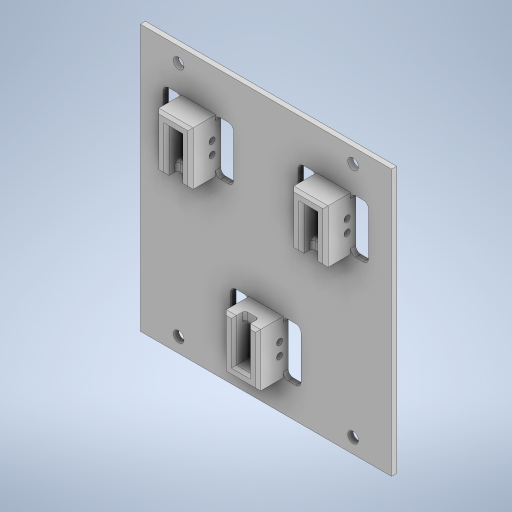
# Autodesk Inventor part: 01EjectionPlate
Saved by Autodesk Inventor 2023 (Build 270158000, 158)
## iProperties
Created: 2023-02-07
Part Number: 01EjectionPlate
Material: Generic
Document SubType Name: Modeling
Designer: 17038
Density: 1 g/cm^3
Appearance: Default
Author: 17038
Autodesk Inventor part; units mm, degrees
ref_plane "YZ Plane" through (0, 0, 0) normal (1, 0, 0) x (0, 1, 0)
ref_plane "XZ Plane" through (0, 0, 0) normal (0, 1, 0) x (-1, 0, 0)
ref_plane "XY Plane" through (0, 0, 0) normal (0, 0, 1) x (1, 0, 0)
sketch "Sketch1" plane through (0, 0, 0) normal (0, 0, 1) x (1, 0, 0)
  line L0 (-49.085, -51.99) -> (49.085, -51.99)
  line L1 (49.085, -51.99) -> (49.085, 51.99)
  line L2 (49.085, 51.99) -> (-49.085, 51.99)
  line L3 (-49.085, 51.99) -> (-49.085, -51.99)
  line L4 (-49.085, -51.99) -> (49.085, 51.99) construction
  line L5 (49.085, -51.99) -> (-49.085, 51.99) construction
  point P0 (0, 0)
  dimension "d0" = 103.98
  dimension "d1" = 98.17
  constraints: 12 end point, 2 midpoint, 2 parallel, 1 horizontal, 1 perpendicular
  measures "d0" distance of L0.end L1.end
  measures "d1" distance of L1.end L2.end
extrude "Extrusion1" add sketch "Sketch1" along normal blind 2
sketch "Sketch2" plane through (0, 0, 2) normal (0, 0, 1) x (1, 0, 0)
  line L0 (49.085, 51.99) -> (-49.085, 51.99) projected
  line L1 (-49.085, 51.99) -> (-49.085, -51.99) projected
  circle A0 centre (-34.085, 46.25) radius 2.05
  line L2 (-49.085, -51.99) -> (49.085, -51.99) construction
  line L3 (0, 51.99) -> (0, -51.99) construction
  circle A1 centre (34.085, 46.25) radius 2.05
  circle A2 centre (-34.085, -46.27) radius 2.05
  circle A3 centre (34.085, -46.27) radius 2.05
  point P0 (0, 0)
  dimension "d4" = 4.1
  dimension "d5" = 5.74
  dimension "d6" = 15
  dimension "d9" = 4.1
  dimension "d10" = 15
  dimension "d11" = 5.72
  constraints: 4 centre point, 2 end point, 2 midpoint, 2 symmetric about line, 2 other
  measures "d4" diameter of A0
  measures "d5" distance from line of L0 A0.centre
  measures "d6" distance from line of L1 A0.centre
  measures "d9" diameter of A2
  measures "d10" distance from line of L1 A2.centre
  measures "d11" distance from line of L2 A2.centre
extrude "Extrusion2" cut sketch "Sketch2" against normal up to surface (2 mm away)
sketch "Sketch4" plane through (0, 0, 2) normal (0, 0, 1) x (1, 0, 0)
  line L0 (49.085, -51.99) -> (49.085, 51.99) projected
  line L1 (49.085, 51.99) -> (-49.085, 51.99) projected
  line L2 (-49.085, 51.99) -> (-49.085, -51.99) projected
  line L3 (-49.085, -51.99) -> (49.085, -51.99) projected
  line L4 (-29.085, 19.19) -> (-23.685, 19.19)
  line L5 (-23.685, 19.19) -> (-23.685, 31.99)
  line L6 (-23.685, 31.99) -> (-29.085, 31.99)
  line L7 (-29.085, 31.99) -> (-29.085, 19.19)
  line L8 (-33.085, 15.19) -> (-19.685, 15.19)
  line L9 (-19.685, 15.19) -> (-19.685, 35.99)
  line L10 (-19.685, 35.99) -> (-33.085, 35.99)
  line L11 (-33.085, 35.99) -> (-33.085, 15.19)
  line L12 (0, 51.99) -> (0, -51.99) construction
  line L13 (29.085, 19.19) -> (23.685, 19.19)
  line L14 (23.685, 19.19) -> (23.685, 31.99)
  line L15 (23.685, 31.99) -> (29.085, 31.99)
  line L16 (29.085, 31.99) -> (29.085, 19.19)
  line L17 (33.085, 15.19) -> (19.685, 15.19)
  line L18 (19.685, 15.19) -> (19.685, 35.99)
  line L19 (19.685, 35.99) -> (33.085, 35.99)
  line L20 (33.085, 35.99) -> (33.085, 15.19)
  line L21 (-49.085, 0) -> (49.085, 0) construction
  line L22 (-2.7, -35.8497) -> (2.7, -35.8497)
  line L23 (2.7, -35.8497) -> (2.7, -23.0497)
  line L24 (2.7, -23.0497) -> (-2.7, -23.0497)
  line L25 (-2.7, -23.0497) -> (-2.7, -35.8497)
  line L26 (-2.7, -35.8497) -> (2.7, -23.0497) construction
  line L27 (2.7, -35.8497) -> (-2.7, -23.0497) construction
  line L28 (-6.7, -39.8497) -> (6.7, -39.8497)
  line L29 (6.7, -39.8497) -> (6.7, -19.0497)
  line L30 (6.7, -19.0497) -> (-6.7, -19.0497)
  line L31 (-6.7, -19.0497) -> (-6.7, -39.8497)
  line L32 (-6.7, -39.8497) -> (6.7, -19.0497) construction
  line L33 (6.7, -39.8497) -> (-6.7, -19.0497) construction
  point P0 (0, 0)
  point P1 (-26.385, 19.19)
  point P2 (0, -29.4497)
  dimension "d12" = 5.4
  dimension "d13" = 12.8
  dimension "d14" = 20
  dimension "d15" = 20
  dimension "d16" = 4
  dimension "d17" = 4
  dimension "d18" = 4
  dimension "d19" = 4
  dimension "d20" = 12.8
  dimension "d21" = 5.4
  dimension "d22" = 4
  dimension "d23" = 4
  dimension "d24" = 4
  dimension "d25" = 4
  constraints: 60 end point, 9 midpoint, 8 parallel, 8 symmetric about line, 4 horizontal, 4 perpendicular, 1 point on line
  measures "d12" distance of L4.start L4.end
  measures "d13" distance of L4.end L5.end
  measures "d14" distance between parallel lines of L1 L6
  measures "d15" distance between parallel lines of L2 L7
  measures "d16" distance between parallel lines of L10 L6
  measures "d17" distance from line of point (-26.385, 19.19) L8
  measures "d18" distance between parallel lines of L11 L7
  measures "d19" distance between parallel lines of L9 L5
  measures "d20" distance of L22.end L23.end
  measures "d21" distance of L23.end L24.end
  measures "d22" distance between parallel lines of L24 L30
  measures "d23" distance between parallel lines of L28 L22
  measures "d24" distance between parallel lines of L31 L25
  measures "d25" distance between parallel lines of L29 L23
extrude "Extrusion3" add sketch "Sketch4" along normal blind 8 contours L11 L10 L9 L8 | L17 L18 L19 L20 | L31 L30 L29 L28
sketch "Sketch5" plane through (0, 0, 2) normal (0, 0, 1) x (1, 0, 0)
  line L0 (-29.085, 19.19) -> (-23.685, 19.19) projected
  line L1 (-23.685, 19.19) -> (-23.685, 31.99) projected
  line L2 (-23.685, 31.99) -> (-29.085, 31.99) projected
  line L3 (-29.085, 31.99) -> (-29.085, 19.19) projected
  line L4 (29.085, 19.19) -> (29.085, 31.99) projected
  line L5 (29.085, 31.99) -> (23.685, 31.99) projected
  line L6 (23.685, 31.99) -> (23.685, 19.19) projected
  line L7 (23.685, 19.19) -> (29.085, 19.19) projected
  line L8 (-2.7, -35.8497) -> (2.7, -35.8497) projected
  line L9 (2.7, -35.8497) -> (2.7, -23.0497) projected
  line L10 (2.7, -23.0497) -> (-2.7, -23.0497) projected
  line L11 (-2.7, -23.0497) -> (-2.7, -35.8497) projected
  point P0 (0, 0)
extrude "Extrusion4" cut sketch "Sketch5" against normal up to surface (2 mm away)
sketch "Sketch6" plane through (0, 0, 10) normal (0, 0, 1) x (1, 0, 0)
  line L0 (-33.085, 15.19) -> (-19.685, 15.19) projected
  line L1 (-23.685, 31.99) -> (-23.685, 19.19) projected
  line L2 (-23.685, 19.19) -> (-29.085, 19.19) projected
  line L3 (19.685, 35.99) -> (19.685, 15.19) projected
  line L4 (19.685, 15.19) -> (33.085, 15.19) projected
  line L5 (33.085, 15.19) -> (33.085, 35.99) projected
  line L6 (33.085, 35.99) -> (19.685, 35.99) projected
  line L7 (29.085, 19.19) -> (23.685, 19.19) projected
  line L8 (23.685, 19.19) -> (23.685, 31.99) projected
  line L9 (23.685, 31.99) -> (29.085, 31.99) projected
  line L10 (29.085, 31.99) -> (29.085, 19.19) projected
  line L11 (6.7, -39.8497) -> (6.7, -19.0497) projected
  line L12 (6.7, -19.0497) -> (-6.7, -19.0497) projected
  line L13 (-6.7, -19.0497) -> (-6.7, -39.8497) projected
  line L14 (-6.7, -39.8497) -> (6.7, -39.8497) projected
  line L15 (-2.7, -35.8497) -> (-2.7, -23.0497) projected
  line L16 (-2.7, -23.0497) -> (2.7, -23.0497) projected
  line L17 (2.7, -23.0497) -> (2.7, -35.8497) projected
  line L18 (2.7, -35.8497) -> (-2.7, -35.8497) projected
  line L19 (-29.085, 19.19) -> (-23.685, 19.19)
  line L20 (-23.685, 19.19) -> (-23.685, 15.19)
  line L21 (-23.685, 15.19) -> (-29.085, 15.19)
  line L22 (-29.085, 15.19) -> (-29.085, 19.19)
  line L23 (23.685, 19.19) -> (29.085, 19.19)
  line L24 (29.085, 19.19) -> (29.085, 15.19)
  line L25 (29.085, 15.19) -> (23.685, 15.19)
  line L26 (23.685, 15.19) -> (23.685, 19.19)
  line L27 (2.7, -23.0997) -> (-2.7, -23.0997) projected
  line L28 (-6.7, -19.0497) -> (6.7, -19.0497) projected
  line L29 (-2.7, -23.0497) -> (2.7, -23.0497)
  line L30 (2.7, -23.0497) -> (2.7, -19.0497)
  line L31 (2.7, -19.0497) -> (-2.7, -19.0497)
  line L32 (-2.7, -19.0497) -> (-2.7, -23.0497)
  point P0 (0, 0)
  point P1 (29.085, 17.19)
  dimension "d30" = 0
  dimension "d31" = 0
  dimension "d32" = 0
  constraints: 24 end point, 6 parallel, 3 horizontal, 3 perpendicular, 3 point on line, 1 midpoint, 1 other
  measures "d30" distance between parallel lines of L1 L20
  measures "d31" distance from line of L10 point (29.085, 17.19)
  measures "d32" distance between parallel lines of L17 L30
extrude "Extrusion5" cut sketch "Sketch6" against normal blind 2.5 contours L22 L2 L20 L0 | L26 L7 L24 L4 | L30 L16 L32 L12
fillet "Fillet1" radius 1 9 edges at (-29.085, 17.19, 7.5) (-23.685, 17.19, 7.5) (29.085, 17.19, 7.5) (23.685, 17.19, 7.5) (-2.7, -21.0497, 7.5) (2.7, -21.0497, 7.5) (0, -23.0497, 7.5) (-26.385, 19.19, 7.5) (26.385, 19.19, 7.5)
sketch "Sketch7" plane through (33.085, 15.19, 2) normal (1, 0, 0) x (0, 0, -1)
  line L0 (0, 0) -> (-8, 0) projected
  circle A0 centre (-1.4, 7.95) radius 1.175
  line L1 (-8, 19.8) -> (-8, 1) projected
  circle A1 centre (-1.4, 12.75) radius 1.175
  point P0 (-7, 0)
  point P1 (2, -15.19)
  dimension "d39" = 2.35
  dimension "d40" = 7.95
  dimension "d41" = 6.6
  dimension "d42" = 2.35
  dimension "d43" = 0
  dimension "d44" = 4.8
  constraints: 2 centre point
  measures "d39" diameter of A0
  measures "d40" distance from line of L0 A0.centre
  measures "d41" distance from line of L1 A0.centre
  measures "d42" diameter of A1
  measures "d43" horizontal distance of A0.centre A1.centre
  measures "d44" distance of A0.centre A1.centre
extrude "Extrusion6" cut sketch "Sketch7" against normal up to surface (66.17 mm away)
sketch "Sketch8" plane through (6.7, -39.8497, 2) normal (1, 0, 0) x (0, 0, -1)
  line L0 (0, 20.8) -> (-8, 20.8) projected
  circle A0 centre (-1.4, 12.85) radius 1.175
  line L1 (-8, 19.8) -> (-8, 1) projected
  line L2 (-8, 1) -> (-7, 0) projected
  line L3 (-7, 0) -> (-7, 20.8) projected
  line L4 (-8, 19.8) -> (-7, 20.8) projected
  circle A1 centre (-1.4, 8.05) radius 1.175
  point P0 (2, 39.8497)
  dimension "d47" = 2.35
  dimension "d48" = 6.6
  dimension "d49" = 7.95
  dimension "d50" = 2.35
  dimension "d51" = 0
  dimension "d52" = 4.8
  constraints: 2 centre point
  measures "d47" diameter of A0
  measures "d48" distance from line of L1 A0.centre
  measures "d49" distance from line of L0 A0.centre
  measures "d50" diameter of A1
  measures "d51" horizontal distance of A0.centre A1.centre
  measures "d52" distance of A0.centre A1.centre
extrude "Extrusion7" cut sketch "Sketch8" against normal up to surface (13.4 mm away) contours A0 | A1
sketch "Sketch9" plane through (0, 0, 2) normal (0, 0, 1) x (1, 0, 0)
  line L0 (49.085, 51.99) -> (-49.085, 51.99) projected
  line L1 (-49.085, -51.99) -> (49.085, -51.99) projected
  line L2 (-19.685, 15.19) -> (-33.085, 15.19) projected
  line L3 (-33.085, 15.19) -> (-33.085, 35.99) projected
  line L4 (-33.085, 35.99) -> (-19.685, 35.99) projected
  line L5 (-19.685, 35.99) -> (-19.685, 15.19) projected
  line L6 (33.085, 35.99) -> (33.085, 15.19) projected
  line L7 (19.685, 15.19) -> (19.685, 35.99) projected
  line L8 (-6.7, -39.8497) -> (-6.7, -19.0497) projected
  line L9 (-6.7, -19.0497) -> (6.7, -19.0497) projected
  line L10 (6.7, -19.0497) -> (6.7, -39.8497) projected
  line L11 (6.7, -39.8497) -> (13.7, -39.8497)
  line L12 (13.7, -39.8497) -> (13.7, -19.0497)
  line L13 (13.7, -19.0497) -> (6.7, -19.0497)
  line L14 (6.7, -19.0497) -> (6.7, -39.8497)
  line L15 (-6.7, -39.8497) -> (-13.7, -39.8497)
  line L16 (-13.7, -39.8497) -> (-13.7, -19.0497)
  line L17 (-13.7, -19.0497) -> (-6.7, -19.0497)
  line L18 (-6.7, -19.0497) -> (-6.7, -39.8497)
  line L19 (-19.685, 15.19) -> (-12.685, 15.19)
  line L20 (-12.685, 15.19) -> (-12.685, 35.99)
  line L21 (-12.685, 35.99) -> (-19.685, 35.99)
  line L22 (-19.685, 35.99) -> (-19.685, 15.19)
  line L23 (-33.085, 35.99) -> (-40.085, 35.99)
  line L24 (-40.085, 35.99) -> (-40.085, 15.19)
  line L25 (-40.085, 15.19) -> (-33.085, 15.19)
  line L26 (-33.085, 15.19) -> (-33.085, 35.99)
  line L27 (0, -51.99) -> (0, 51.99) construction
  line L28 (33.085, 15.19) -> (33.085, 35.99)
  line L29 (19.685, 15.19) -> (12.685, 15.19)
  line L30 (12.685, 15.19) -> (12.685, 35.99)
  line L31 (12.685, 35.99) -> (19.685, 35.99)
  line L32 (19.685, 35.99) -> (19.685, 15.19)
  line L33 (33.085, 35.99) -> (40.085, 35.99)
  line L34 (40.085, 35.99) -> (40.085, 15.19)
  line L35 (40.085, 15.19) -> (33.085, 15.19)
  point P0 (0, 0)
  point P1 (-6.7, -19.0497)
  dimension "d55" = 0
  dimension "d56" = 0
  dimension "d57" = 0
  dimension "d58" = 7
  dimension "d59" = 7
  dimension "d60" = 7
  dimension "d61" = 7
  constraints: 50 end point, 8 parallel, 7 symmetric about line, 4 horizontal, 4 perpendicular, 2 midpoint, 1 point on line
  measures "d55" distance between parallel lines of L2 L25
  measures "d56" distance between parallel lines of L9 L13
  measures "d57" distance between parallel lines of L4 L21
  measures "d58" distance between parallel lines of L10 L12
  measures "d59" distance between parallel lines of L18 L16
  measures "d60" distance between parallel lines of L5 L20
  measures "d61" distance between parallel lines of L3 L24
extrude "Extrusion8" cut sketch "Sketch9" against normal up to surface (2 mm away) contours L5 L21 L20 L19 | L25 L24 L23 L3 | L33 L34 L35 L6 | L29 L30 L31 L7 | L15 L16 L17 L8 | L13 L12 L11 L10
fillet "Fillet2" radius 2 24 edges at (-19.685, 15.19, 1) (-12.685, 15.19, 1) (-12.685, 35.99, 1) (-19.685, 35.99, 1) (-33.085, 15.19, 1) (-40.085, 15.19, 1) (-40.085, 35.99, 1) (-33.085, 35.99, 1) (19.685, 35.99, 1) (40.085, 35.99, 1) (13.7, -19.0497, 1) (12.685, 15.19, 1) (12.685, 35.99, 1) (19.685, 15.19, 1) (33.085, 15.19, 1) (40.085, 15.19, 1) (33.085, 35.99, 1) (6.7, -19.0497, 1) (6.7, -39.8497, 1) (13.7, -39.8497, 1) (-6.7, -39.8497, 1) (-13.7, -39.8497, 1) (-13.7, -19.0497, 1) (-6.7, -19.0497, 1)
sketch "Sketch13" plane through (0, 0, 10) normal (0, 0, 1) x (1, 0, 0)
  line L0 (-1.7, -23.0497) -> (1.7, -23.0497) projected
  line L1 (-2.7, -23.0497) -> (-1.7, -23.0497) projected
  line L2 (-2.7, -35.8497) -> (-2.7, -19.0497) projected
  line L3 (1.7, -23.0497) -> (2.7, -23.0497) projected
  line L4 (2.7, -19.0497) -> (2.7, -35.8497) projected
  line L5 (2.7, -35.8497) -> (-2.7, -35.8497) projected
  line L6 (-24.685, 19.19) -> (-28.085, 19.19) projected
  line L7 (-23.685, 31.99) -> (-23.685, 15.19) projected
  line L8 (-24.685, 18.19) -> (-24.685, 19.19) projected
  line L9 (-23.685, 19.19) -> (-24.685, 19.19) projected
  line L10 (-28.085, 19.19) -> (-29.085, 19.19) projected
  line L11 (-29.085, 15.19) -> (-29.085, 31.99) projected
  line L12 (-29.085, 31.99) -> (-23.685, 31.99) projected
  line L13 (28.085, 19.19) -> (24.685, 19.19) projected
  line L14 (29.085, 19.19) -> (28.085, 19.19) projected
  line L15 (24.685, 19.19) -> (23.685, 19.19) projected
  line L16 (23.685, 15.19) -> (23.685, 31.99) projected
  line L17 (29.085, 31.99) -> (29.085, 15.19) projected
  line L18 (23.685, 31.99) -> (29.085, 31.99) projected
  point P0 (0, 0)
extrude "Extrusion12" cut sketch "Sketch13" against normal up to surface (10 mm away)
sketch "Sketch15" plane through (0, 0, 10) normal (0, 0, 1) x (1, 0, 0)
  line L0 (-23.685, 31.99) -> (-23.685, 15.19) projected
  line L1 (-23.685, 15.19) -> (-19.685, 15.19) projected
  line L2 (-19.685, 15.19) -> (-19.685, 35.99) projected
  line L3 (-19.685, 35.99) -> (-33.085, 35.99) projected
  line L4 (-33.085, 35.99) -> (-33.085, 15.19) projected
  line L5 (-33.085, 15.19) -> (-29.085, 15.19) projected
  line L6 (-29.085, 15.19) -> (-29.085, 31.99) projected
  line L7 (-29.085, 31.99) -> (-23.685, 31.99) projected
  line L8 (29.085, 31.99) -> (29.085, 15.19) projected
  line L9 (29.085, 15.19) -> (33.085, 15.19) projected
  line L10 (33.085, 15.19) -> (33.085, 35.99) projected
  line L11 (33.085, 35.99) -> (19.685, 35.99) projected
  line L12 (19.685, 35.99) -> (19.685, 15.19) projected
  line L13 (19.685, 15.19) -> (23.685, 15.19) projected
  line L14 (23.685, 15.19) -> (23.685, 31.99) projected
  line L15 (23.685, 31.99) -> (29.085, 31.99) projected
  line L16 (2.7, -19.0497) -> (2.7, -35.8497) projected
  line L17 (2.7, -35.8497) -> (-2.7, -35.8497) projected
  line L18 (-2.7, -35.8497) -> (-2.7, -19.0497) projected
  line L19 (-2.7, -19.0497) -> (-6.7, -19.0497) projected
  line L20 (-6.7, -19.0497) -> (-6.7, -39.8497) projected
  line L21 (-6.7, -39.8497) -> (6.7, -39.8497) projected
  line L22 (6.7, -39.8497) -> (6.7, -19.0497) projected
  line L23 (6.7, -19.0497) -> (2.7, -19.0497) projected
  point P0 (0, 0)
extrude "Extrusion13" add sketch "Sketch15" along normal blind 1.8
chamfer "Chamfer2" distance 1 angle 45 24 edges at (-29.085, 23.59, 11.8) (-33.085, 25.59, 11.8) (-26.385, 35.99, 11.8) (-26.385, 31.99, 11.8) (-23.685, 23.59, 11.8) (-19.685, 25.59, 11.8) (-21.685, 15.19, 11.8) (-31.085, 15.19, 11.8) (19.685, 25.59, 11.8) (26.385, 35.99, 11.8) (23.685, 23.59, 11.8) (26.385, 31.99, 11.8) (29.085, 23.59, 11.8) (33.085, 25.59, 11.8) (31.085, 15.19, 11.8) (21.685, 15.19, 11.8) (4.7, -19.0497, 11.8) (6.7, -29.4497, 11.8) (2.7, -27.4497, 11.8) (0, -35.8497, 11.8) (-2.7, -27.4497, 11.8) (-6.7, -29.4497, 11.8) (-4.7, -19.0497, 11.8) (0, -39.8497, 11.8)
equation "\"d9\" = d4"
equation "\"d10\" = d6"
equation "\"d42\" = d39"
equation "\"d48\" = d41"
equation "\"d49\" = d40"
equation "\"d50\" = d47"
equation "\"d52\" = d44"
body "Solid1"
